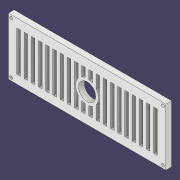
# Autodesk Inventor part: HA006
Saved by Autodesk Inventor 2017 SP1 (Build 210196100, 196)
## iProperties
Created: 2017-06-25
Part Number: HA006
Material: ABS Plastic
Document SubType Name: Modeling
Designer: Zach
Density: 1.06 g/cm^3
Appearance: CR White
Author: Zach
Autodesk Inventor part; units mm, degrees
ref_plane "YZ Plane" through (0, 0, 0) normal (1, 0, 0) x (0, 1, 0)
ref_plane "XZ Plane" through (0, 0, 0) normal (0, 1, 0) x (-1, 0, 0)
ref_plane "XY Plane" through (0, 0, 0) normal (0, 0, 1) x (1, 0, 0)
sketch "Sketch1" plane through (0, 0, 0) normal (0, 0, 1) x (1, 0, 0)
  line L0 (0, 0) -> (275, 0)
  line L1 (275, 0) -> (275, 100)
  line L2 (275, 100) -> (0, 100)
  line L3 (0, 100) -> (0, 0)
  dimension "d0" = 275
  dimension "d1" = 100
  constraints: 8 end point, 2 parallel, 1 horizontal, 1 perpendicular
  measures "d0" distance of L2.end L1.end
  measures "d1" distance of L1.end L0.end
extrude "Extrusion1" add sketch "Sketch1" along normal blind 10
sketch "Sketch2" plane through (0, 0, 10) normal (0, 0, 1) x (1, 0, 0)
  line L0 (0, 0) -> (275, 0) construction
  line L1 (275, 0) -> (275, 100) construction
  line L2 (275, 100) -> (0, 100) construction
  line L3 (0, 100) -> (0, 0) construction
  line L4 (5, 95) -> (270, 95) construction
  line L5 (270, 95) -> (270, 5) construction
  line L6 (270, 5) -> (5, 5) construction
  line L7 (5, 5) -> (5, 95) construction
  line L8 (10, 90) -> (265, 90) construction
  line L9 (265, 90) -> (265, 10) construction
  line L10 (265, 10) -> (10, 10) construction
  line L11 (10, 10) -> (10, 90) construction
  circle A0 centre (5, 95) radius 2.5
  circle A1 centre (270, 95) radius 2.5
  circle A2 centre (270, 5) radius 2.5
  circle A3 centre (5, 5) radius 2.5
  line L12 (15, 85) -> (21, 85)
  line L13 (21, 85) -> (21, 15)
  line L14 (21, 15) -> (15, 15)
  line L15 (15, 15) -> (15, 85)
  line L16 (15, 85) -> (260, 85) construction
  line L17 (260, 85) -> (260, 15) construction
  line L18 (260, 15) -> (15, 15) construction
  line L19 (15, 15) -> (15, 85) construction
  line L20 (33.57, 85) -> (33.57, 15)
  line L21 (27.57, 85) -> (33.57, 85)
  line L22 (27.57, 15) -> (27.57, 85)
  line L23 (27.57, 15) -> (27.57, 85) construction
  line L24 (33.57, 15) -> (27.57, 15)
  line L25 (46.14, 85) -> (46.14, 15)
  line L26 (40.14, 85) -> (46.14, 85)
  line L27 (40.14, 15) -> (40.14, 85)
  line L28 (40.14, 15) -> (40.14, 85) construction
  line L29 (46.14, 15) -> (40.14, 15)
  line L30 (58.71, 85) -> (58.71, 15)
  line L31 (52.71, 85) -> (58.71, 85)
  line L32 (52.71, 15) -> (52.71, 85)
  line L33 (52.71, 15) -> (52.71, 85) construction
  line L34 (58.71, 15) -> (52.71, 15)
  line L35 (71.28, 85) -> (71.28, 15)
  line L36 (65.28, 85) -> (71.28, 85)
  line L37 (65.28, 15) -> (65.28, 85)
  line L38 (65.28, 15) -> (65.28, 85) construction
  line L39 (71.28, 15) -> (65.28, 15)
  line L40 (83.85, 85) -> (83.85, 15)
  line L41 (77.85, 85) -> (83.85, 85)
  line L42 (77.85, 15) -> (77.85, 85)
  line L43 (77.85, 15) -> (77.85, 85) construction
  line L44 (83.85, 15) -> (77.85, 15)
  line L45 (96.42, 85) -> (96.42, 15)
  line L46 (90.42, 85) -> (96.42, 85)
  line L47 (90.42, 15) -> (90.42, 85)
  line L48 (90.42, 15) -> (90.42, 85) construction
  line L49 (96.42, 15) -> (90.42, 15)
  line L50 (108.99, 85) -> (108.99, 15)
  line L51 (102.99, 85) -> (108.99, 85)
  line L52 (102.99, 15) -> (102.99, 85)
  line L53 (102.99, 15) -> (102.99, 85) construction
  line L54 (108.99, 15) -> (102.99, 15)
  line L55 (121.56, 85) -> (121.56, 15)
  line L56 (115.56, 85) -> (121.56, 85)
  line L57 (115.56, 15) -> (115.56, 85)
  line L58 (115.56, 15) -> (115.56, 85) construction
  line L59 (121.56, 15) -> (115.56, 15)
  line L60 (134.13, 85) -> (134.13, 15)
  line L61 (128.13, 85) -> (134.13, 85)
  line L62 (128.13, 15) -> (128.13, 85)
  line L63 (128.13, 15) -> (128.13, 85) construction
  line L64 (134.13, 15) -> (128.13, 15)
  line L65 (146.7, 85) -> (146.7, 15)
  line L66 (140.7, 85) -> (146.7, 85)
  line L67 (140.7, 15) -> (140.7, 85)
  line L68 (140.7, 15) -> (140.7, 85) construction
  line L69 (146.7, 15) -> (140.7, 15)
  line L70 (159.27, 85) -> (159.27, 15)
  line L71 (153.27, 85) -> (159.27, 85)
  line L72 (153.27, 15) -> (153.27, 85)
  line L73 (153.27, 15) -> (153.27, 85) construction
  line L74 (159.27, 15) -> (153.27, 15)
  line L75 (171.84, 85) -> (171.84, 15)
  line L76 (165.84, 85) -> (171.84, 85)
  line L77 (165.84, 15) -> (165.84, 85)
  line L78 (165.84, 15) -> (165.84, 85) construction
  line L79 (171.84, 15) -> (165.84, 15)
  line L80 (184.41, 85) -> (184.41, 15)
  line L81 (178.41, 85) -> (184.41, 85)
  line L82 (178.41, 15) -> (178.41, 85)
  line L83 (178.41, 15) -> (178.41, 85) construction
  line L84 (184.41, 15) -> (178.41, 15)
  line L85 (196.98, 85) -> (196.98, 15)
  line L86 (190.98, 85) -> (196.98, 85)
  line L87 (190.98, 15) -> (190.98, 85)
  line L88 (190.98, 15) -> (190.98, 85) construction
  line L89 (196.98, 15) -> (190.98, 15)
  line L90 (209.55, 85) -> (209.55, 15)
  line L91 (203.55, 85) -> (209.55, 85)
  line L92 (203.55, 15) -> (203.55, 85)
  line L93 (203.55, 15) -> (203.55, 85) construction
  line L94 (209.55, 15) -> (203.55, 15)
  line L95 (222.12, 85) -> (222.12, 15)
  line L96 (216.12, 85) -> (222.12, 85)
  line L97 (216.12, 15) -> (216.12, 85)
  line L98 (216.12, 15) -> (216.12, 85) construction
  line L99 (222.12, 15) -> (216.12, 15)
  line L100 (234.69, 85) -> (234.69, 15)
  line L101 (228.69, 85) -> (234.69, 85)
  line L102 (228.69, 15) -> (228.69, 85)
  line L103 (228.69, 15) -> (228.69, 85) construction
  line L104 (234.69, 15) -> (228.69, 15)
  line L105 (247.26, 85) -> (247.26, 15)
  line L106 (241.26, 85) -> (247.26, 85)
  line L107 (241.26, 15) -> (241.26, 85)
  line L108 (241.26, 15) -> (241.26, 85) construction
  line L109 (247.26, 15) -> (241.26, 15)
  line L110 (259.83, 85) -> (259.83, 15)
  line L111 (253.83, 85) -> (259.83, 85)
  line L112 (253.83, 15) -> (253.83, 85)
  line L113 (253.83, 15) -> (253.83, 85) construction
  line L114 (259.83, 15) -> (253.83, 15)
  dimension "d4" = 5
  dimension "d5" = 10
  dimension "d6" = 5
  dimension "d7" = 5
  dimension "d8" = 5
  dimension "d9" = 5
  dimension "d10" = 6
  dimension "d11" = 15
  dimension "d14" = 12.57
  constraints: 222 end point, 4 centre point, 4 coincident, 2 horizontal, 2 parallel, 1 perpendicular, 1 point on line, 199 other
  measures "d4" distance between parallel lines of L2 L4
  measures "d5" distance between parallel lines of L2 L8
  measures "d6" diameter of A0
  measures "d7" diameter of A1
  measures "d8" diameter of A2
  measures "d9" diameter of A3
  measures "d10" distance of L14.end L13.end
  measures "d11" distance between parallel lines of L2 L16
  measures "d14" distance of L12.end L20.start
extrude "Extrusion2" cut sketch "Sketch2" against normal through all
sketch "Sketch4" plane through (0, 0, 10) normal (0, 0, 1) x (1, 0, 0)
  circle A0 centre (137.5, 50) radius 15
  line L0 (275, 100) -> (0, 100) projected
  line L1 (275, 0) -> (275, 100) projected
  point P0 (0, 0)
  point P1 (275, 50)
  point P2 (137.5, 100)
  dimension "d23" = 30
  constraints: 2 midpoint, 1 centre point, 1 horizontal alignment, 1 vertical alignment
  measures "d23" diameter of A0
extrude "Extrusion4" cut sketch "Sketch4" against normal through all
sketch "Sketch5" plane through (0, 0, 10) normal (0, 0, 1) x (1, 0, 0)
  arc A0 (140.7, 64.6547) -> (134.13, 64.6165) centre (137.5, 50) ccw projected
  circle A1 centre (137.5, 50) radius 15
  circle A2 centre (137.5, 50) radius 20
  point P0 (0, 0)
  dimension "d26" = 5
  constraints: 1 centre point, 1 coincident, 3 other
extrude "Extrusion5" add sketch "Sketch5" against normal blind 10
body "Solid1"
